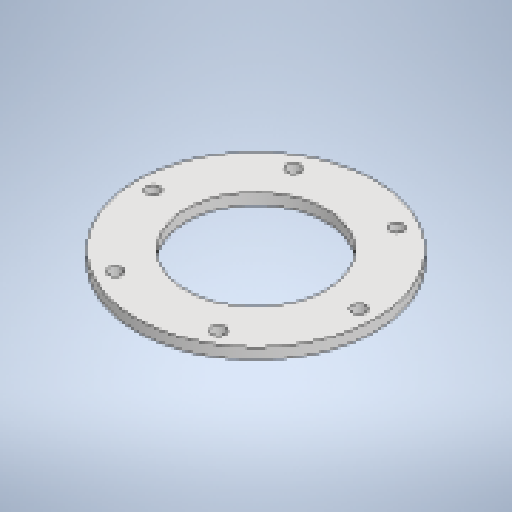
# Autodesk Inventor part: NVPH-402 tube flange 1
Saved by Autodesk Inventor 2025.1 (Build 291241020, 241B)
## iProperties
Created: 2024-12-03
Part Number: NVPH-402 tube flange 1
Material: Generic
Document SubType Name: Sheet Metal
Designer: user
Density: 1 g/cm^3
Appearance: Default
Sheet Metal Rule: Default_mm
Author: user
Autodesk Inventor part; units mm, degrees
ref_plane "YZ Plane" through (0, 0, 0) normal (1, 0, 0) x (0, 1, 0)
ref_plane "XZ Plane" through (0, 0, 0) normal (0, 1, 0) x (-1, 0, 0)
ref_plane "XY Plane" through (0, 0, 0) normal (0, 0, 1) x (1, 0, 0)
sketch "Sketch1" plane through (0, 0, 0) normal (0, 0, 1) x (1, 0, 0)
  circle A0 centre (0, 0) radius 63
  circle A1 centre (0, 0) radius 107.5
  dimension "d0" = 126
  dimension "d1" = 215
  constraints: 2 centre point, 2 coincident
  measures "d0" diameter of A0
  measures "d1" diameter of A1
extrude "Extrusion1" add sketch "Sketch1" against normal blind 10
sketch "Sketch3" plane through (0, 0, 0) normal (0, 0, 1) x (1, 0, 0)
  circle A0 centre (92.5, 0) radius 6
  circle A1 centre (0, 0) radius 92.5 construction
  dimension "d4" = 185
  dimension "d5" = 12
  constraints: 2 horizontal alignment, 1 centre point, 1 coincident, 2 other
  measures "d5" diameter of A0
extrude "Cut1" cut sketch "Sketch3" against normal blind 10
pattern_circular "Circular Pattern1" count 6 over 360 about axis through (0, 0, 0) along (0, 0, -1) of "Cut1"
equation "\"d4\" = back_steel_circle_диам_центров"
equation "\"d7\" = Thickness"
equation "\"BendReliefDepth\" = 0.5 * Thickness"
equation "\"back_steel_circle_диам_центров\" = 185"
equation "\"Thickness\" = 10"
body "Solid1"
